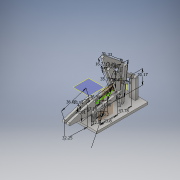
# Autodesk Inventor part: body
Saved by Autodesk Inventor 2016 (Build 200138000, 138)
## iProperties
Created: 2018-05-06
Part Number: body
Material: 一般
Document SubType Name: Modeling
Designer: 黃胤瑋
Density: 1 g/cm^3
Appearance: 預設
Author: 黃胤瑋
Autodesk Inventor part; units mm, degrees
ref_plane "YZ Plane" through (0, 0, 0) normal (1, 0, 0) x (0, 1, 0)
ref_plane "XZ Plane" through (0, 0, 0) normal (0, 1, 0) x (-1, 0, 0)
ref_plane "XY Plane" through (0, 0, 0) normal (0, 0, 1) x (1, 0, 0)
sketch "草圖1" plane through (0, 0, 0) normal (1, 0, 0) x (0, 1, 0)
  line L0 (0, 6) -> (-10.6691, 0.7747)
  line L1 (0, 12.8) -> (-21.6115, 15.7356)
  line L2 (-9.9069, 17.9378) -> (-21.6115, 15.7356)
  line L3 (-9.9069, 17.9378) -> (-10.8826, 50.173)
  line L4 (-10.8826, 50.173) -> (-21.6115, 15.7356)
  line L5 (-15.9576, -18.5134) -> (-48.9584, -6.411)
  line L6 (-48.9584, -6.411) -> (-36.3559, -18.2482)
  line L7 (-36.3559, -18.2482) -> (-15.9576, -18.5134)
  line L8 (-48.9584, -6.411) -> (-64.7968, -1.0222)
  line L9 (-64.7968, -1.0222) -> (-41.8907, -29.2211)
  line L10 (-41.8907, -29.2211) -> (-48.9584, -6.411)
  line L11 (-41.8907, -29.2211) -> (0, -23.8)
  line L12 (-15.9576, -18.5134) -> (-10.4, -10.2)
  line L13 (-36.3559, -18.2482) -> (-20.17, -43.78)
  line L14 (-15.9576, -18.5134) -> (-10.6691, 0.7747)
  line L15 (-9.9069, 17.9378) -> (-10.6691, 0.7747)
  line L16 (-9.9069, 17.9378) -> (-15.9576, -18.5134)
  point P0 (0, 0)
  dimension "d1" = 11.88
  dimension "d2" = 21.81
  dimension "d4" = 36.95
  dimension "d5" = 11.91
  dimension "d6" = 32.25
  dimension "d7" = 36.07
  dimension "d8" = 35.15
  dimension "d9" = 6
  dimension "d10" = 10.2
  dimension "d11" = 10.4
  dimension "d13" = 20.4
  dimension "d14" = 17.29
  dimension "d15" = 23.8
  dimension "d16" = 42.24
  dimension "d18" = 23.88
  dimension "d19" = 36.33
  dimension "d20" = 16.73
  dimension "d22" = 20.17
  dimension "d23" = 43.78
  dimension "d24" = 30.23
  dimension "d25" = 10
  dimension "d26" = 20
  dimension "d105" = 17.18
  dimension "d166" = 12.8
  constraints: 34 end point, 3 vertical alignment
  measures "d1" distance of L0.start L0.end
  measures "d2" distance of L1.end L1.start
  measures "d4" distance of L5.start L2.start
  measures "d5" distance of L2.start L1.end
  measures "d6" distance of L2.start L3.end
  measures "d7" distance of L3.end L1.end
  measures "d8" distance of L5.start L5.end
  measures "d9" distance of point (0, 0) L0.start
  measures "d10" vertical distance of point (0, 0) L12.end
  measures "d11" horizontal distance of point (0, 0) L12.end
  measures "d13" distance of L6.end L5.start
  measures "d14" distance of L5.end L6.end
  measures "d15" distance of point (0, 0) L11.end
  measures "d16" distance of L9.end L11.end
  measures "d18" distance of L9.end L5.end
  measures "d19" distance of L8.end L9.end
  measures "d20" distance of L5.end L8.end
  measures "d22" horizontal distance of point (0, 0) L13.end
  measures "d23" vertical distance of point (0, 0) L13.end
  measures "d24" distance of L6.end L13.end
  measures "d25" distance of L5.start L12.end
  measures "d26" distance of L5.start L0.end
  measures "d105" distance of L2.start L0.end
  measures "d166" distance of point (0, 0) L1.start
sketch "草圖4" plane through (0, 0, 0) normal (1, 0, 0) x (0, 1, 0)
  line L0 (-48.2698, -4.5333) -> (-15.269, -16.6357)
  line L1 (-15.9836, -20.5133) -> (-36.3819, -20.2481)
  line L2 (-37.7251, -19.706) -> (-50.3277, -7.8688)
  arc A0 (-48.2698, -4.5333) -> (-50.3277, -7.8688) centre (-48.9584, -6.411) ccw
  arc A1 (-37.7251, -19.706) -> (-36.3819, -20.2481) centre (-36.3559, -18.2482) ccw
  arc A2 (-15.9836, -20.5133) -> (-15.269, -16.6357) centre (-15.9576, -18.5134) ccw
  circle A3 centre (-15.9576, -18.5134) radius 1
  circle A4 centre (-48.9584, -6.411) radius 1
  circle A5 centre (-36.3559, -18.2482) radius 1
  point P0 (0, 0)
  point P1 (-27.8274, -17.6895)
  dimension "d35" = 2
  dimension "d36" = 2
  dimension "d37" = 2
  dimension "d38" = 2
  constraints: 6 centre point, 6 coincident, 6 end point, 6 point on circle, 6 tangent, 2 equal radius
  measures "d35" radius of A0
  measures "d36" diameter of A3
  measures "d37" diameter of A4
  measures "d38" diameter of A5
extrude "擠出1" add sketch "草圖4" along normal mid plane 3
sketch "草圖5" plane through (-1.5, 0, 0) normal (-1, 0, 0) x (0, 0, 1)
  circle A0 centre (-18.5134, -15.9576) radius 1
  circle A1 centre (-10.2, -10.4) radius 1
  line L0 (-18.5134, -15.9576) -> (-10.2, -10.4) construction
  line L1 (-17.4019, -17.6203) -> (-9.0885, -12.0627)
  line L2 (-11.3115, -8.7373) -> (-19.6249, -14.2949)
  arc A2 (-19.6249, -14.2949) -> (-17.4019, -17.6203) centre (-18.5134, -15.9576) ccw
  arc A3 (-9.0885, -12.0627) -> (-11.3115, -8.7373) centre (-10.2, -10.4) ccw
  point P0 (0, 0)
  point P1 (-14.3567, -13.1788)
  dimension "d41" = 2
  dimension "d42" = 2
  dimension "d43" = 1
  constraints: 8 end point, 4 centre point, 4 point on circle, 4 tangent, 2 coincident, 1 midpoint, 1 parallel
  measures "d41" diameter of A1
  measures "d42" diameter of A0
  measures "d43" radial gap between concentric circles of A1 A3
extrude "擠出2" add sketch "草圖5" along normal blind 3 separate body
sketch "草圖6" plane through (-1.5, 0, 0) normal (-1, 0, 0) x (0, 0, 1)
  line L0 (-18.2482, -36.3559) -> (-43.78, -20.17) construction
  line L1 (-17.1774, -34.6667) -> (-42.7092, -18.4808)
  line L2 (-44.8508, -21.8592) -> (-19.3191, -38.045)
  arc A0 (-19.3191, -38.045) -> (-17.1774, -34.6667) centre (-18.2482, -36.3559) ccw
  arc A1 (-42.7092, -18.4808) -> (-44.8508, -21.8592) centre (-43.78, -20.17) ccw
  circle A2 centre (-43.78, -20.17) radius 1
  circle A3 centre (-18.2482, -36.3559) radius 1
  point P0 (0, 0)
  point P1 (-31.0141, -28.2629)
  dimension "d46" = 2
  dimension "d47" = 2
  dimension "d48" = 1
  constraints: 8 end point, 4 centre point, 4 point on circle, 4 tangent, 2 coincident, 1 midpoint, 1 parallel
  measures "d46" diameter of A3
  measures "d47" diameter of A2
  measures "d48" radial gap between concentric circles of A2 A1
extrude "擠出3" add sketch "草圖6" along normal blind 3 separate body
sketch "草圖7" plane through (0, 0, 0) normal (1, 0, 0) x (0, 1, 0)
  circle A0 centre (0, -23.8) radius 1
  circle A1 centre (-41.8907, -29.2211) radius 1
  line L0 (-41.8907, -29.2211) -> (0, -23.8) construction
  line L1 (-42.1474, -27.2377) -> (-0.2567, -21.8165)
  line L2 (0.2567, -25.7835) -> (-41.634, -31.2046)
  arc A2 (-42.1474, -27.2377) -> (-41.634, -31.2046) centre (-41.8907, -29.2211) ccw
  arc A3 (0.2567, -25.7835) -> (-0.2567, -21.8165) centre (0, -23.8) ccw
  point P0 (0, 0)
  point P1 (-20.9453, -26.5106)
  dimension "d51" = 2
  dimension "d52" = 2
  dimension "d53" = 1
  constraints: 8 end point, 4 centre point, 4 point on circle, 4 tangent, 2 coincident, 1 midpoint, 1 parallel
  measures "d51" diameter of A0
  measures "d52" diameter of A1
  measures "d53" radial gap between concentric circles of A1 A2
extrude "擠出4" add sketch "草圖7" along normal mid plane 3 separate body
ref_plane "工作平面1" through (-3, 0, 0) normal (-1, 0, 0) x (0, 0, 1)
mirror "鏡射1" about plane through (-3, 0, 0) normal (-1, 0, 0) bodies 1 separate body
sketch "草圖8" plane through (-3, 0, 0) normal (-1, 0, 0) x (0, 0, 1)
  line L0 (-2.2832, -66.3492) -> (-30.4821, -43.4431)
  line L1 (-28.6292, -39.9803) -> (-5.8191, -47.048)
  line L2 (-4.5176, -48.3142) -> (0.8712, -64.1526)
  arc A0 (-2.2832, -66.3492) -> (0.8712, -64.1526) centre (-1.0222, -64.7968) ccw
  arc A1 (-4.5176, -48.3142) -> (-5.8191, -47.048) centre (-6.411, -48.9584) ccw
  arc A2 (-28.6292, -39.9803) -> (-30.4821, -43.4431) centre (-29.2211, -41.8907) ccw
  circle A3 centre (-1.0222, -64.7968) radius 1
  circle A4 centre (-6.411, -48.9584) radius 1
  circle A5 centre (-29.2211, -41.8907) radius 1 projected
  circle A6 centre (-29.2211, -41.8907) radius 1
  point P0 (0, 0)
  dimension "d57" = 2
  dimension "d58" = 2
  dimension "d59" = 2
  dimension "d60" = 2
  constraints: 6 centre point, 6 coincident, 6 end point, 6 point on circle, 6 tangent, 2 equal radius
  measures "d57" radius of A0
  measures "d58" diameter of A6
  measures "d59" diameter of A3
  measures "d60" diameter of A4
extrude "擠出5" add sketch "草圖8" along normal mid plane 3 separate body
mirror "鏡射2" about plane through (-3, 0, 0) normal (-1, 0, 0) bodies 4 separate body
sketch "草圖12" plane through (-1.5, 0, 0) normal (-1, 0, 0) x (0, 0, 1)
  circle A0 centre (6, 0) radius 1
  circle A1 centre (0.7747, -10.6691) radius 1
  line L0 (0.7747, -10.6691) -> (6, 0) construction
  line L1 (2.5709, -11.5488) -> (7.7962, -0.8797)
  line L2 (4.2038, 0.8797) -> (-1.0214, -9.7895)
  arc A2 (-1.0214, -9.7895) -> (2.5709, -11.5488) centre (0.7747, -10.6691) ccw
  arc A3 (7.7962, -0.8797) -> (4.2038, 0.8797) centre (6, 0) ccw
  point P0 (0, 0)
  point P1 (3.3874, -5.3346)
  dimension "d74" = 2
  dimension "d75" = 2
  dimension "d76" = 1
  constraints: 8 end point, 4 centre point, 4 point on circle, 4 tangent, 2 coincident, 1 midpoint, 1 parallel
  measures "d74" diameter of A0
  measures "d75" diameter of A1
  measures "d76" radial gap between concentric circles of A0 A3
extrude "擠出9" add sketch "草圖12" along normal blind 3 separate body
sketch "草圖15" plane through (-1.5, 0, 0) normal (-1, 0, 0) x (0, 0, 1)
  circle A0 centre (12.8, 0) radius 1
  circle A1 centre (15.7356, -21.6115) radius 1
  line L0 (15.7356, -21.6115) -> (12.8, 0) construction
  line L1 (17.7174, -21.3423) -> (14.7818, 0.2692)
  line L2 (10.8182, -0.2692) -> (13.7538, -21.8807)
  arc A2 (13.7538, -21.8807) -> (17.7174, -21.3423) centre (15.7356, -21.6115) ccw
  arc A3 (14.7818, 0.2692) -> (10.8182, -0.2692) centre (12.8, 0) ccw
  point P0 (0, 0)
  point P1 (14.2678, -10.8058)
  dimension "d86" = 2
  dimension "d87" = 2
  dimension "d88" = 1
  constraints: 8 end point, 4 centre point, 4 point on circle, 4 tangent, 2 coincident, 1 midpoint, 1 parallel
  measures "d86" diameter of A1
  measures "d87" diameter of A0
  measures "d88" radial gap between concentric circles of A0 A3
extrude "擠出12" add sketch "草圖15" along normal blind 3 separate body
sketch "草圖17" plane through (-1.5, 0, 0) normal (1, 0, 0) x (0, 0, -1)
  line L0 (-16.3305, -23.521) -> (-50.7679, -12.7921)
  line L1 (-50.2335, -8.8835) -> (-17.9983, -7.9078)
  line L2 (-15.9723, -9.5371) -> (-13.7701, -21.2417)
  arc A0 (-16.3305, -23.521) -> (-13.7701, -21.2417) centre (-15.7356, -21.6115) ccw
  arc A1 (-15.9723, -9.5371) -> (-17.9983, -7.9078) centre (-17.9378, -9.9069) ccw
  arc A2 (-50.2335, -8.8835) -> (-50.7679, -12.7921) centre (-50.173, -10.8826) ccw
  circle A3 centre (-15.7356, -21.6115) radius 1 projected
  circle A4 centre (-15.7356, -21.6115) radius 1
  circle A5 centre (-17.9378, -9.9069) radius 1
  circle A6 centre (-50.173, -10.8826) radius 1
  point P0 (0, 0)
  dimension "d97" = 2
  dimension "d98" = 2
  dimension "d99" = 2
  dimension "d100" = 2
  constraints: 6 centre point, 6 coincident, 6 end point, 6 point on circle, 6 tangent, 2 equal radius
  measures "d97" radius of A0
  measures "d98" diameter of A6
  measures "d99" diameter of A5
  measures "d100" diameter of A4
extrude "擠出14" add sketch "草圖17" along normal blind 3 separate body
mirror "鏡射3" about plane through (-3, 0, 0) normal (-1, 0, 0) bodies 10 separate body
sketch "草圖19" plane through (1.5, 0, 0) normal (1, 0, 0) x (0, 0, -1)
  line L0 (18.1859, -17.9306) -> (-18.2653, -11.8799)
  line L1 (-17.8491, -7.9089) -> (-0.686, -8.6711)
  line L2 (-0.2459, -8.7403) -> (19.0423, -14.0288)
  arc A0 (18.1859, -17.9306) -> (19.0423, -14.0288) centre (18.5134, -15.9576) ccw
  arc A1 (-17.8491, -7.9089) -> (-18.2653, -11.8799) centre (-17.9378, -9.9069) ccw
  arc A2 (-0.2459, -8.7403) -> (-0.686, -8.6711) centre (-0.7747, -10.6691) ccw
  circle A3 centre (18.5134, -15.9576) radius 1 projected
  circle A4 centre (18.5134, -15.9576) radius 1
  circle A5 centre (-17.9378, -9.9069) radius 1 projected
  circle A6 centre (-17.9378, -9.9069) radius 1
  dimension "d107" = 2
  dimension "d108" = 2
  constraints: 6 end point, 6 point on circle, 6 tangent, 5 centre point, 5 coincident, 1 equal radius
  measures "d107" radius of A0
  measures "d108" radius of A2
extrude "擠出16" add sketch "草圖19" along normal blind 3 separate body
mirror "鏡射4" about plane through (-3, 0, 0) normal (-1, 0, 0) bodies 12 separate body
move or copy body "移動本體1" bodies to move or copy 8 copy no translate (-3, 0, 0)
mirror "鏡射5" about plane through (-3, 0, 0) normal (-1, 0, 0) bodies 8 separate body
sketch "草圖22" plane through (-3, 0, 0) normal (-1, 0, 0) x (0, 0, 1)
  circle A0 centre (6, 0) radius 2
  circle A1 centre (-23.8, 0) radius 1 projected
  circle A2 centre (-23.8, 0) radius 2
  point P0 (0, 0)
  point P1 (12.8, 0)
  dimension "d117" = 4
  dimension "d118" = 4
  constraints: 2 centre point, 2 coincident
  measures "d117" diameter of A0
  measures "d118" diameter of A2
extrude "擠出18" add sketch "草圖22" along normal mid plane 3 separate body
sketch "草圖24" plane through (-3, 0, 0) normal (-1, 0, 0) x (0, 0, 1)
  circle A0 centre (6, 0) radius 2 projected
  circle A1 centre (-23.8, 0) radius 2 projected
  line L0 (6, 0) -> (4, 0)
  line L1 (4.5, 6.3553) -> (6, 6.3553)
  line L2 (6, 6.3553) -> (6, 0)
  line L3 (4.5, 0) -> (4.5, 6.3553)
  point P0 (0, 0)
  dimension "d159" = 3
  constraints: 8 end point, 1 horizontal, 1 horizontal alignment, 1 parallel, 1 perpendicular, 1 point on line, 1 other
  measures "d159" diameter of L3 L2
revolve "迴轉1" add sketch "草圖24" angle 360 about axis through (-3, 6.3553, 6) along (0, -1, 0) bodies 15 contours L3 L1 L2 A0 | A0 L2 L0 L3
sketch "草圖25" plane through (-3, 0, 0) normal (-1, 0, 0) x (0, 0, 1)
  circle A0 centre (-23.8, 0) radius 2 projected
  line L0 (-23.8, 0) -> (-25.3, 0)
  line L1 (-25.3, 6.3553) -> (-23.8, 6.3553)
  line L2 (-23.8, 6.3553) -> (-23.8, 0)
  line L3 (7.5, 6.3553) -> (4.5, 6.3553) projected
  line L4 (-25.3, 0) -> (-25.3, 6.3553)
  point P0 (0, 0)
  point P1 (-25.8, 0)
  dimension "d160" = 3
  constraints: 8 end point, 2 horizontal alignment, 1 horizontal, 1 parallel, 1 perpendicular, 1 other
  measures "d160" diameter of L4 L2
revolve "迴轉2" add sketch "草圖25" angle 360 about axis through (-3, 6.3553, -23.8) along (0, -1, 0) picked at (-24.8, 0.441) bodies 15 contours L2 L0 L4 A0 | A0 L4 L1 L2
ref_plane "工作平面3" through (-7.5, 0, 0) normal (-1, 0, 0) x (0, 0, 1)
sketch "草圖31" plane through (-7.5, 0, 0) normal (-1, 0, 0) x (0, 0, 1)
  line L0 (-9.2, -10.4) -> (-11.2, -10.4) projected
  arc A0 (-11.2, -10.4) -> (-9.2, -10.4) centre (-10.2, -10.4) ccw projected
  arc A1 (-12.2, -10.4) -> (-8.2, -10.4) centre (-10.2, -10.4) ccw projected
  line L1 (-8.2, -10.4) -> (-8.2, 6.3553) projected
  line L2 (-8.2, 6.3553) -> (-12.2, 6.3553) projected
  line L3 (-12.2, 6.3553) -> (-12.2, -10.4) projected
  circle A2 centre (-10.2, -10.4) radius 1
  point P0 (0, 0)
  constraints: 1 coincident, 1 horizontal alignment, 2 other
extrude "擠出24" cut sketch "草圖31" against normal blind 9 contours L0 A2 bodies 3 15
sketch "草圖32" plane through (-3, 0, 0) normal (-1, 0, 0) x (0, 0, 1)
  arc A0 (-12.2, -10.4) -> (-8.2, -10.4) centre (-10.2, -10.4) ccw projected
  line L0 (-12.2, -10.4) -> (-12.2, 6.3553) projected
  line L1 (-12.2, 6.3553) -> (-8.2, 6.3553) projected
  line L2 (-8.2, 6.3553) -> (-8.2, -10.4) projected
  circle A1 centre (-10.2, -10.4) radius 1 projected
  line L3 (-8.2, -8.4) -> (-12.2, -8.4)
  line L4 (-12.2, -10.4) -> (-12.2, 6.3553) projected
  circle A2 centre (-10.2, -10.4) radius 2
  line L5 (-8.2, -8.4) -> (-8.2, -10.4)
  line L6 (-12.2, -8.4) -> (-12.2, -10.4)
  point P0 (0, 0)
  constraints: 6 end point, 5 point on circle, 3 tangent, 2 point on line, 1 centre point, 1 coincident, 1 horizontal
extrude "擠出25" cut sketch "草圖32" along normal mid plane 3 contours A2 A0 | L0 L3 A2 | A2 L3 L2 bodies 3 15
sketch "草圖33" plane through (-4.5, 0, 0) normal (-1, 0, 0) x (0, 0, 1)
  arc A0 (-42.7092, -18.4808) -> (-44.8508, -21.8592) centre (-43.78, -20.17) ccw projected
  circle A1 centre (-43.78, -20.17) radius 2
  line L0 (-41.78, -20.17) -> (-45.78, -20.17)
  line L1 (-45.78, -20.17) -> (-45.78, 6.3553)
  line L2 (-45.78, 6.3553) -> (-41.78, 6.3553)
  line L3 (-41.78, 6.3553) -> (-41.78, -20.17)
  line L4 (-22.3, 6.3553) -> (-25.3, 6.3553) projected
  point P0 (0, 0)
  constraints: 8 end point, 3 point on circle, 2 horizontal alignment, 2 parallel, 1 centre point, 1 coincident, 1 horizontal, 1 perpendicular
extrude "擠出26" add sketch "草圖33" along normal blind 3 and the other way blind 6 bodies 15
sketch "草圖34" plane through (-7.5, 0, 0) normal (-1, 0, 0) x (0, 0, 1)
  arc A0 (-45.78, -20.17) -> (-41.78, -20.17) centre (-43.78, -20.17) ccw projected
  line L0 (-41.78, -20.17) -> (-41.78, 6.3553) projected
  line L1 (-41.78, 6.3553) -> (-45.78, 6.3553) projected
  line L2 (-45.78, 6.3553) -> (-45.78, -20.17) projected
  circle A1 centre (-43.78, -20.17) radius 1
  point P0 (0, 0)
  dimension "d142" = 2
  constraints: 1 centre point, 1 coincident
  measures "d142" diameter of A1
extrude "擠出27" cut sketch "草圖34" against normal through all contours A1 bodies 3 15
sketch "草圖35" plane through (-3, 0, 0) normal (-1, 0, 0) x (0, 0, 1)
  circle A0 centre (-43.78, -20.17) radius 1 projected
  arc A1 (-45.78, -20.17) -> (-41.78, -20.17) centre (-43.78, -20.17) ccw projected
  line L0 (-45.78, -20.17) -> (-45.78, 6.3553) projected
  line L1 (-45.78, 6.3553) -> (-41.78, 6.3553) projected
  line L2 (-41.78, 6.3553) -> (-41.78, -20.17) projected
  circle A2 centre (-43.78, -20.17) radius 2
  line L3 (-41.78, -18.17) -> (-45.78, -18.17)
  line L4 (-45.78, -18.17) -> (-45.78, -20.17)
  line L5 (-41.78, -18.17) -> (-41.78, -20.17)
  point P0 (0, 0)
  constraints: 6 end point, 4 point on circle, 3 tangent, 2 point on line, 1 centre point, 1 coincident, 1 concentric, 1 perpendicular
extrude "擠出28" cut sketch "草圖35" along normal mid plane 3 contours A2 A1 | L0 L3 A2 | A2 L3 L2 bodies 15
ref_plane "工作平面2" through (-7.5, 6.3553, -12.2) normal (0, 1, 0) x (1, 0, 0)
sketch "草圖36" plane through (-7.5, 6.3553, -12.2) normal (0, 1, 0) x (1, 0, 0)
  line L0 (-10.5, -35.4) -> (19.5, -35.4)
  line L1 (19.5, -35.4) -> (19.5, 36.6)
  line L2 (19.5, 36.6) -> (-10.5, 36.6)
  line L3 (-10.5, 36.6) -> (-10.5, -35.4)
  circle A0 centre (4.5, 11.6) radius 1.5 projected
  point P0 (7.5, -12.2)
  dimension "d147" = 30
  dimension "d148" = 15
  dimension "d149" = 72
  dimension "d150" = 25
  constraints: 8 end point, 2 parallel, 1 horizontal, 1 perpendicular
  measures "d147" distance of L1.end L2.end
  measures "d148" distance from line of L3 A0.centre
  measures "d149" distance of L2.end L0.start
  measures "d150" distance from line of A0.centre L2
extrude "擠出29" add sketch "草圖36" along normal blind 3 contours L3 L2 L1 L0 | A0 bodies 15
sketch "草圖37" plane through (-3, 0, 0) normal (-1, 0, 0) x (0, 0, 1)
  circle A0 centre (6, 0) radius 1 projected
  circle A1 centre (-23.8, 0) radius 1 projected
  point P0 (0, 0)
extrude "擠出30" cut sketch "草圖37" against normal through all bodies 3 15
sketch "草圖38" plane through (-7.5, -42.1474, -27.2377) normal (-1, 0, 0) x (0, -0.1283414, 0.9917301)
  circle A0 centre (-2, 42.24) radius 1 projected
  point P0 (21.6032, 45.2945)
extrude "擠出31" cut sketch "草圖38" against normal blind 30 bodies 7 15
sketch "草圖39" plane through (-7.5, -11.5488, 2.5709) normal (-1, 0, 0) x (0, -0.4398391, 0.8980766)
  circle A0 centre (-2, 11.88) radius 1 projected
  point P0 (-7.3885, 9.241)
extrude "擠出32" cut sketch "草圖39" against normal blind 30 bodies 15
sketch "草圖40" plane through (-3, 0, 0) normal (-1, 0, 0) x (0, 0, 1)
  arc A0 (14.7818, 0.2692) -> (10.8182, -0.2692) centre (12.8, 0) ccw projected
  circle A1 centre (12.8, 0) radius 2
  line L0 (11.2472, -3.4272) -> (15.2108, -2.8888)
  line L1 (17.7174, -21.3423) -> (14.7818, 0.2692) projected
  line L2 (10.8182, -0.2692) -> (13.7538, -21.8807) projected
  point P0 (0, 0)
  dimension "d161" = 90
  constraints: 2 end point, 2 point on line, 1 coincident, 3 other
  measures "d161" angle of L1 L0
extrude "擠出33" cut sketch "草圖40" along normal mid plane 1.5 bodies 3 9
sketch "草圖41" plane through (-3, 0, 0) normal (-1, 0, 0) x (0, 0, 1)
  arc A0 (14.7818, 0.2692) -> (10.8182, -0.2692) centre (12.8, 0) ccw projected
  arc A1 (10.8, 0) -> (14.8, 0) centre (12.8, 0) ccw
  line L0 (10.8, 0) -> (10.8, 7.1661)
  line L1 (10.8, 7.1661) -> (14.8, 7.1661)
  line L2 (14.8, 7.1661) -> (14.8, 0)
  line L3 (23.2, 6.3553) -> (-48.8, 6.3553) projected
  circle A2 centre (12.8, 0) radius 1 projected
  point P0 (0, 0)
  constraints: 6 end point, 3 point on circle, 1 centre point, 1 coincident, 1 concentric, 1 parallel
extrude "擠出34" add sketch "草圖41" along normal mid plane 1.5 bodies 15
sketch "草圖42" plane through (-10.5, -17.9306, -18.1859) normal (-1, 0, 0) x (0, 0.1637539, 0.9865012)
  circle A0 centre (36.95, 2) radius 1 projected
  circle A1 centre (0, 2) radius 1 projected
  line L0 (-0.2059, 3.9894) -> (19.6879, 6.0479) projected
  arc A2 (-0.2059, 3.9894) -> (0, 0) centre (0, 2) ccw projected
  line L1 (36.95, 0) -> (0, 0) projected
  arc A3 (36.95, 0) -> (37.1896, 3.9856) centre (36.95, 2) ccw projected
  line L2 (20.1334, 6.0441) -> (37.1896, 3.9856) projected
  arc A4 (20.1334, 6.0441) -> (19.6879, 6.0479) centre (19.8938, 4.0586) ccw projected
  circle A5 centre (19.8938, 4.0586) radius 1 projected
  point P0 (20.8766, 14.7105)
extrude "擠出35" cut sketch "草圖42" against normal through all contours A5 bodies 13 12
sketch "草圖43" plane through (-3, 0, 0) normal (-1, 0, 0) x (0, 0, 1)
  circle A0 centre (-10.2, -10.4) radius 1 projected
  circle A1 centre (-18.5134, -15.9576) radius 1 projected
  line L0 (-17.4019, -17.6203) -> (-9.0885, -12.0627) projected
  arc A2 (-19.6249, -14.2949) -> (-17.4019, -17.6203) centre (-18.5134, -15.9576) ccw projected
  line L1 (-11.3115, -8.7373) -> (-19.6249, -14.2949) projected
  arc A3 (-9.0885, -12.0627) -> (-11.3115, -8.7373) centre (-10.2, -10.4) ccw projected
  line L2 (-17.4019, -17.6203) -> (-9.0885, -12.0627) projected
  circle A4 centre (-10.2, -10.4) radius 2
  line L3 (-13.2452, -14.8415) -> (-15.4682, -11.5161)
  line L4 (-11.3115, -8.7373) -> (-19.6249, -14.2949) projected
  point P0 (0, 0)
  dimension "d169" = 5
  constraints: 2 end point, 2 midpoint, 1 coincident, 1 perpendicular, 3 other
  measures "d169" distance from line of A0.centre L3
extrude "擠出36" cut sketch "草圖43" along normal mid plane 1.5 contours L3 L1 A4 L0 | A4 A3 bodies 3
move or copy body "移動本體2" bodies to move or copy 2 copy no translate (9, 0, 0)
sketch "草圖47" plane through (7.5, -12.0627, -9.0885) normal (1, 0, 0) x (0, -0.8313428, 0.55576)
  circle A0 centre (-2, 0) radius 1 projected
  arc A1 (-0.8885, -1.6627) -> (-3.1115, 1.6627) centre (-2, 0) ccw
  line L0 (-37.3818, 22.7779) -> (2.633, -37.0788) projected
  line L1 (-3.1115, 1.6627) -> (-17.0409, -7.6493)
  line L2 (-0.8885, -1.6627) -> (-14.8179, -10.9746)
  line L3 (2.633, -37.0788) -> (-37.3818, 22.7779) projected
  line L4 (-17.0409, -7.6493) -> (-14.8179, -10.9746)
  point P0 (-4.9772, -14.2596)
  point P1 (-3.9006, -0.6226)
  point P2 (13.2365, -52.9402)
  dimension "d182" = 4
  dimension "d185" = 90
  constraints: 6 end point, 3 point on circle, 3 point on line, 2 tangent, 1 centre point, 1 coincident, 1 collinear, 1 perpendicular
  measures "d182" diameter of A1
  measures "d185" angle of L0 L2
extrude "擠出39" add sketch "草圖47" along normal blind 3 bodies 15
